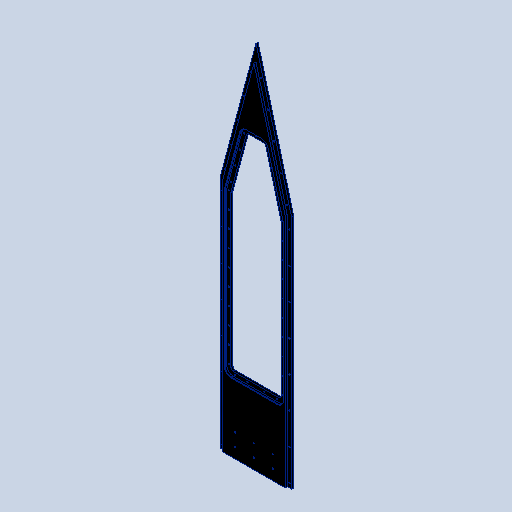
# Autodesk Inventor part: Model Shell_part1_side_plate
Saved by Autodesk Inventor 2023 (Build 270158000, 158)
## iProperties
Created: 2022-12-13
Part Number: Model Shell_part1_side_plate
Material: Aluminum 6061
Document SubType Name: Modeling
Designer: Tanzu
Density: 2.7 g/cm^3
Appearance: White
Mass: 6356.21 g
Surface Area: 9912.85 cm^2
Volume: 2354.15 cm^3
Author: Tanzu
Autodesk Inventor part; units mm, degrees
(part 1 of 2)
ref_plane "YZ Plane" through (0, 0, 0) normal (1, 0, 0) x (0, 1, 0)
ref_plane "XZ Plane" through (0, 0, 0) normal (0, 1, 0) x (-1, 0, 0)
ref_plane "XY Plane" through (0, 0, 0) normal (0, 0, 1) x (1, 0, 0)
sketch "Sketch2" plane through (0, 0, 0) normal (0, 0, 1) x (1, 0, 0)
  line L0 (-90, 0) -> (90, 0) construction
  line L1 (90, 0) -> (90, 900) construction
  line L2 (90, 900) -> (-90, 900) construction
  line L3 (-90, 900) -> (-90, 0) construction
  line L4 (-90, 250) -> (90, 250) construction
  line L5 (0, 900) -> (90, 564.1154)
  line L6 (0, 900) -> (-90, 564.1154)
  line L7 (0, 900) -> (0, 250) construction
  line L8 (-132.5, 0) -> (132.5, 0) construction
  line L9 (-90, 564.1154) -> (-90, 0)
  line L10 (90, 564.1154) -> (90, 0)
  line L11 (90, 0) -> (-90, 0)
  line L12 (-85, 563.4572) -> (0, 880.6815)
  line L13 (0, 880.6815) -> (85, 563.4572)
  line L14 (85, 563.4572) -> (85, 5)
  line L15 (85, 5) -> (-85, 5)
  line L16 (-85, 5) -> (-85, 563.4572)
  line L17 (-85, 5) -> (-85, 0)
  line L18 (85, 5) -> (85, 0)
  line L19 (40, 731.3995) -> (-40, 731.3995)
  line L20 (90, 564.1154) -> (-90, 564.1154) construction
  line L21 (85, 563.4572) -> (85, 564.1154)
  line L22 (85, 564.1154) -> (84.8236, 564.1154)
  line L23 (-85, 563.4572) -> (-85, 564.1154)
  line L24 (-85, 564.1154) -> (-84.8236, 564.1154)
  point P0 (0, 0)
  point P1 (0, 0)
  dimension "d4" = 180
  dimension "d5" = 900
  dimension "d6" = 250
  dimension "d7" = 15
  dimension "d8" = 15
  dimension "d9" = 265
  dimension "d10" = 5
  dimension "d265" = 80
  constraints: 50 end point, 15 point on line, 6 perpendicular, 4 midpoint, 3 coincident, 3 collinear, 2 horizontal, 2 parallel, 4 other
  measures "d4" distance of L0.start L0.end
  measures "d5" distance of L0.end L1.end
  measures "d6" distance between parallel lines of L0 L4
  measures "d7" angle of L7 L5
  measures "d8" angle of L6 L7
  measures "d9" distance of L8.start L8.end
  measures "d10" distance between parallel lines of L6 L12
  measures "d265" distance of L19.start L19.end
extrude "Extrusion2" add sketch "Sketch2" along normal mid plane 180
sketch "Sketch3" plane through (0, 0, 0) normal (0, 0, 1) x (1, 0, 0)
  line L0 (-132.5, 0) -> (132.5, 0)
  line L1 (-90, 0) -> (90, 0) projected
  line L2 (0, 0) -> (0, 600)
  line L3 (0, 600) -> (-132.5, 0)
  line L4 (0, 601.0824) -> (0, 600)
  line L5 (0, 577.3585) -> (-127.5, 0)
  line L6 (0, 577.3585) -> (0, 601.0824)
  point P0 (0, 0)
  dimension "d13" = 265
  dimension "d14" = 600
  dimension "d17" = 5
  constraints: 12 end point, 3 point on line, 2 midpoint, 2 vertical, 1 collinear, 1 horizontal, 1 parallel
  measures "d13" distance of L0.start L0.end
  measures "d14" distance of L2.start L2.end
  measures "d17" distance of L0.start L5.end
revolve "Revolution1" [suppressed]
revolve "Revolution2" [suppressed]
extrude "Extrusion3" cut sketch "Sketch2" along normal mid plane 160 contours L11 L17 L15 L18 | L15 L16 L12 L19 L13 L14 | L13 L22 L21 | L23 L24 L12 | L19 L12 L13
sketch "Sketch5" plane through (0, 0, 0) normal (0, -1, 0) x (1, 0, 0)
  circle A0 centre (0, 0) radius 127.5 projected
  circle A1 centre (0, 0) radius 132.5 projected
extrude "Extrusion4" [suppressed]
fillet "Fillet1" [suppressed]
sketch "Sketch6" plane through (90, 564.1154, 90) normal (1, 0, 0) x (0, 0, -1)
  line L0 (180, 0) -> (180, -564.1154) projected
  line L1 (180, 0) -> (0, 0) projected
  line L2 (0, -564.1154) -> (0, 0) projected
  line L3 (27.5, -275) -> (152.5, -275)
  line L4 (152.5, -275) -> (152.5, -75)
  line L5 (152.5, -75) -> (27.5, -75)
  line L6 (27.5, -75) -> (27.5, -275)
  line L7 (180, -564.1154) -> (0, -564.1154) projected
  point P0 (90, -564.1154)
  point P1 (90, 0)
  point P2 (90, -75)
  dimension "d25" = 75
  dimension "d26" = 200
  dimension "d27" = 125
  constraints: 8 end point, 2 midpoint, 2 parallel, 1 horizontal, 1 perpendicular, 1 vertical alignment
  measures "d25" distance between parallel lines of L1 L5
  measures "d26" distance of L5.end L3.start
  measures "d27" distance of L3.start L3.end
extrude "Extrusion5" cut sketch "Sketch6" against normal up to next contours L6 L5 L4 L3
sketch "Sketch7" plane through (85, 33.0197, 85) normal (-1, 0, 0) x (0, 0, 1)
  line L0 (-22.5, 256.0957) -> (-22.5, 456.0957) projected
  line L1 (-147.5, 256.0957) -> (-22.5, 256.0957) projected
  line L2 (-147.5, 456.0957) -> (-147.5, 256.0957) projected
  line L3 (-22.5, 456.0957) -> (-147.5, 456.0957) projected
  line L4 (-32.5, 446.0957) -> (-32.5, 266.0957)
  line L5 (-32.5, 266.0957) -> (-137.5, 266.0957)
  line L6 (-137.5, 266.0957) -> (-137.5, 446.0957)
  line L7 (-137.5, 446.0957) -> (-32.5, 446.0957)
  point P0 (-85, -33.0197)
  dimension "d30" = 10
  constraints: 8 end point, 3 other
  measures "d30" distance between parallel lines of L0 L4
extrude "Extrusion6" [suppressed]
fillet "Fillet3" radius 5 4 edges at (87.5, 289.1154, 62.5) (87.5, 289.1154, -62.5) (87.5, 489.1154, 62.5) (87.5, 489.1154, -62.5)
sketch "Sketch8" plane through (0, 0, -90) normal (0, 0, -1) x (-1, 0, 0)
  line L0 (90, 0) -> (90, 564.1154) projected
  line L1 (90, 564.1154) -> (0, 900) projected
  line L2 (0, 900) -> (-90, 564.1154) projected
  line L3 (-90, 564.1154) -> (-90, 0) projected
  line L4 (-90, 564.1154) -> (0, 900) projected
  line L5 (-20.0962, 825) -> (20.0962, 825)
  line L6 (0, 900) -> (90, 564.1154) projected
  line L7 (-90, 0) -> (90, 0) projected
  point P0 (0, 0)
  point P1 (20.0962, 825)
  dimension "d34" = 75
  constraints: 2 end point, 2 point on line, 1 horizontal
  measures "d34" distance from line of L1.end L5
extrude "Extrusion7" [suppressed]
sketch "Sketch9" plane through (0, 0, -90) normal (0, 0, -1) x (-1, 0, 0)
  line L0 (0, 900) -> (-90, 564.1154) projected
  line L1 (-90, 564.1154) -> (-90, 0) projected
  line L2 (90, 0) -> (90, 564.1154) projected
  line L3 (90, 564.1154) -> (0, 900) projected
  line L4 (-55, 164.1154) -> (55, 164.1154)
  line L5 (70, 179.1154) -> (70, 542.1406)
  line L6 (70, 544.1154) -> (-70, 544.1154) construction
  line L7 (-70, 542.1406) -> (-70, 179.1154)
  line L8 (-69.4889, 546.0229) -> (-32.7866, 682.9977)
  line L9 (-18.2977, 694.1154) -> (18.2977, 694.1154)
  line L10 (-90, 0) -> (-90, 564.1154) projected
  line L11 (32.7866, 682.9977) -> (69.4889, 546.0229)
  line L12 (-20.0962, 825) -> (-90, 564.1154) projected
  line L13 (90, 564.1154) -> (20.0962, 825) projected
  arc A0 (-70, 179.1154) -> (-55, 164.1154) centre (-55, 179.1154) ccw
  arc A1 (55, 164.1154) -> (70, 179.1154) centre (55, 179.1154) ccw
  arc A2 (-18.2977, 694.1154) -> (-32.7866, 682.9977) centre (-18.2977, 679.1154) ccw
  arc A3 (32.7866, 682.9977) -> (18.2977, 694.1154) centre (18.2977, 679.1154) ccw
  arc A4 (-69.4889, 546.0229) -> (-70, 542.1406) centre (-55, 542.1406) ccw
  arc A5 (70, 542.1406) -> (69.4889, 546.0229) centre (55, 542.1406) ccw
  line L14 (70, 542.1406) -> (70, 544.1154) construction
  line L15 (70, 544.1154) -> (69.4889, 546.0229) construction
  line L16 (-70, 542.1406) -> (-70, 544.1154) construction
  line L17 (-69.4889, 546.0229) -> (-70, 544.1154) construction
  line L18 (-65, 179.1154) -> (-65, 542.1406) construction
  arc A6 (-64.6593, 544.7288) -> (-65, 542.1406) centre (-55, 542.1406) ccw construction
  line L19 (-64.6593, 544.7288) -> (-27.957, 681.7036) construction
  arc A7 (-18.2977, 689.1154) -> (-27.957, 681.7036) centre (-18.2977, 679.1154) ccw construction
  line L20 (-18.2977, 689.1154) -> (18.2977, 689.1154) construction
  arc A8 (27.957, 681.7036) -> (18.2977, 689.1154) centre (18.2977, 679.1154) ccw construction
  line L21 (27.957, 681.7036) -> (64.6593, 544.7288) construction
  arc A9 (65, 542.1406) -> (64.6593, 544.7288) centre (55, 542.1406) ccw construction
  line L22 (65, 542.1406) -> (65, 179.1154) construction
  arc A10 (55, 169.1154) -> (65, 179.1154) centre (55, 179.1154) ccw construction
  line L23 (55, 169.1154) -> (-55, 169.1154) construction
  arc A11 (-65, 179.1154) -> (-55, 169.1154) centre (-55, 179.1154) ccw construction
  line L24 (-60, 542.1406) -> (-60, 179.1154)
  arc A12 (-60, 179.1154) -> (-55, 174.1154) centre (-55, 179.1154) ccw
  line L25 (-55, 174.1154) -> (55, 174.1154)
  arc A13 (55, 174.1154) -> (60, 179.1154) centre (55, 179.1154) ccw
  line L26 (60, 179.1154) -> (60, 542.1406)
  arc A14 (60, 542.1406) -> (59.8296, 543.4347) centre (55, 542.1406) ccw
  line L27 (59.8296, 543.4347) -> (23.1273, 680.4095)
  arc A15 (23.1273, 680.4095) -> (18.2977, 684.1154) centre (18.2977, 679.1154) ccw
  line L28 (18.2977, 684.1154) -> (-18.2977, 684.1154)
  arc A16 (-18.2977, 684.1154) -> (-23.1273, 680.4095) centre (-18.2977, 679.1154) ccw
  line L29 (-23.1273, 680.4095) -> (-59.8296, 543.4347)
  arc A17 (-59.8296, 543.4347) -> (-60, 542.1406) centre (-55, 542.1406) ccw
  circle A18 centre (-65, 184.1154) radius 1.5
  circle A19 centre (65, 184.1154) radius 1.5
  circle A20 centre (-65, 224.1154) radius 1.5
  circle A21 centre (65, 224.1154) radius 1.5
  circle A22 centre (-65, 264.1154) radius 1.5
  circle A23 centre (65, 264.1154) radius 1.5
  circle A24 centre (-65, 304.1154) radius 1.5
  circle A25 centre (65, 304.1154) radius 1.5
  circle A26 centre (-65, 344.1154) radius 1.5
  circle A27 centre (65, 344.1154) radius 1.5
  circle A28 centre (-65, 384.1154) radius 1.5
  circle A29 centre (65, 384.1154) radius 1.5
  circle A30 centre (-65, 424.1154) radius 1.5
  circle A31 centre (65, 424.1154) radius 1.5
  circle A32 centre (-65, 464.1154) radius 1.5
  circle A33 centre (65, 464.1154) radius 1.5
  circle A34 centre (-50, 169.1154) radius 1.5
  circle A35 centre (-20, 169.1154) radius 1.5
  circle A36 centre (-59.4646, 564.1154) radius 1.5
  circle A37 centre (-49.1119, 602.7525) radius 1.5
  circle A38 centre (-38.7591, 641.3895) radius 1.5
  circle A39 centre (-28.4063, 680.0265) radius 1.5
  circle A40 centre (0, 689.1154) radius 1.5
  line L30 (0, 164.1154) -> (0, 174.1154) construction
  circle A41 centre (50, 169.1154) radius 1.5
  circle A42 centre (20, 169.1154) radius 1.5
  circle A43 centre (59.4646, 564.1154) radius 1.5
  circle A44 centre (49.1119, 602.7525) radius 1.5
  circle A45 centre (38.7591, 641.3895) radius 1.5
  circle A46 centre (28.4063, 680.0265) radius 1.5
  line L31 (-90, 0) -> (90, 0) projected
  circle A47 centre (-65, 504.1154) radius 1.5
  circle A48 centre (65, 504.1154) radius 1.5
  circle A49 centre (-65, 544.1154) radius 1.5
  circle A50 centre (65, 544.1154) radius 1.5
  point P0 (0, 0)
  point P1 (-90, 37.1533)
  dimension "d37" = 20
  dimension "d38" = 20
  dimension "d39" = 20
  dimension "d41" = 150
  dimension "d42" = 15
  dimension "d43" = 15
  dimension "d44" = 15
  dimension "d45" = 15
  dimension "d46" = 15
  dimension "d47" = 15
  dimension "d48" = 380
  dimension "d49" = 5
  dimension "d50" = 5
  dimension "d51" = 3
  dimension "d52" = 3
  dimension "d53" = 10
  dimension "d59" = 40
  dimension "d63" = 3
  dimension "d64" = 15
  dimension "d70" = 30
  dimension "d72" = 3
  dimension "d79" = 40
  dimension "d81" = 3
  dimension "d721" = 20
  constraints: 51 centre point, 48 end point, 36 point on circle, 14 tangent, 6 parallel, 6 symmetric about line, 4 perpendicular, 4 point on line, 3 midpoint, 3 vertical, 2 horizontal, 1 collinear, 1 horizontal alignment, 73 other
  measures "d37" distance between parallel lines of L1 L7
  measures "d38" distance between parallel lines of L2 L5
  measures "d39" distance from line of L0.end L6
  measures "d41" distance between parallel lines of L6 L9
  measures "d42" radius of A1
  measures "d43" radius of A0
  measures "d44" radius of A4
  measures "d45" radius of A5
  measures "d46" radius of A2
  measures "d47" radius of A3
  measures "d48" distance between parallel lines of L6 L4
  measures "d49" distance between parallel lines of L7 L18
  measures "d50" distance between parallel lines of L24 L18
  measures "d51" diameter of A18
  measures "d52" diameter of A19
  measures "d53" distance from line of A18.centre L25
  measures "d59" distance of A18.centre A20.centre
  measures "d63" diameter of A34
  measures "d64" distance from line of L18 A34.centre
  measures "d70" distance of A34.centre A35.centre
  measures "d72" diameter of A36
  measures "d79" distance of A36.centre A37.centre
  measures "d81" diameter of A40
  measures "d721" vertical distance of A49.centre A36.centre
extrude "Extrusion8" cut sketch "Sketch9" against normal up to next contours A17 L29 A16 L28 A15 L27 A14 L26 A13 L25 A12 L24 | A18 | A19 | A20 | A21 | A22 | A23 | A24 | A25 | A26 | A27 | A28 | A29 | A30 | A31 | A32 | A33 | A34 | A35 | A36 | A37 | A38 | A39 | A40 | A41 | A42 | A43 | A44 | A45 | A46 | A47 | A48 | A49 | A50
extrude "Extrusion9" cut sketch "Sketch9" against normal blind 5 contours A0 L7 A4 L8 A2 L9 A3 L11 A5 L5 A1 L4 | A47 | A48 | A49 | A50
mirror "Mirror1" about plane through (0, 0, 0) normal (0, 0, 1) of "Extrusion8", "Extrusion9"
sketch "Sketch28" plane through (90, 0, 90) normal (1, 0, 0) x (0, 0, -1)
  arc A0 (147.5, 289.1154) -> (152.5, 294.1154) centre (147.5, 294.1154) ccw projected
  line L0 (147.5, 289.1154) -> (32.5, 289.1154) projected
  line L1 (152.5, 484.1154) -> (152.5, 294.1154) projected
  line L2 (32.5, 489.1154) -> (147.5, 489.1154) projected
  arc A1 (152.5, 484.1154) -> (147.5, 489.1154) centre (147.5, 484.1154) ccw projected
  line L3 (27.5, 294.1154) -> (27.5, 484.1154) projected
  arc A2 (32.5, 489.1154) -> (27.5, 484.1154) centre (32.5, 484.1154) ccw projected
  arc A3 (27.5, 294.1154) -> (32.5, 289.1154) centre (32.5, 294.1154) ccw projected
  line L4 (29.5, 484.1154) -> (29.5, 294.1154)
  arc A4 (29.5, 294.1154) -> (32.5, 291.1154) centre (32.5, 294.1154) ccw
  line L5 (32.5, 291.1154) -> (147.5, 291.1154)
  arc A5 (147.5, 291.1154) -> (150.5, 294.1154) centre (147.5, 294.1154) ccw
  line L6 (150.5, 294.1154) -> (150.5, 484.1154)
  arc A6 (150.5, 484.1154) -> (147.5, 487.1154) centre (147.5, 484.1154) ccw
  line L7 (147.5, 487.1154) -> (32.5, 487.1154)
  arc A7 (32.5, 487.1154) -> (29.5, 484.1154) centre (32.5, 484.1154) ccw
  point P0 (90, 0)
  dimension "d386" = 2
  constraints: 8 end point, 8 point on circle, 4 centre point, 7 other
  measures "d386" radial gap between concentric circles of A2 A7
extrude "Extrusion21" add sketch "Sketch28" along normal blind 2 from surface at -5
chamfer "Chamfer2" distance 1 angle 45 24 edges at (65.6066, 168.5088, -90) (70, 360.628, -90) (69.8717, 544.0985, -90) (51.1377, 614.5103, -90) (27.4291, 691.0157, -90) (0, 694.1154, -90) (-27.4291, 691.0157, -90) (-51.1377, 614.5103, -90) (-69.8717, 544.0985, -90) (-70, 360.628, -90) (-65.6066, 168.5088, -90) (0, 164.1154, -90) (0, 164.1154, 90) (-65.6066, 168.5088, 90) (-70, 360.628, 90) (-69.8717, 544.0985, 90) (-51.1377, 614.5103, 90) (-27.4291, 691.0157, 90) (0, 694.1154, 90) (27.4291, 691.0157, 90) (51.1377, 614.5103, 90) (69.8717, 544.0985, 90) (70, 360.628, 90) (65.6066, 168.5088, 90)
sketch "Sketch18" plane through (0, 0, 0) normal (0, 1, 0) x (-1, 0, 0)
  line L0 (-85, 80) -> (85, 80)
  line L1 (85, 80) -> (85, -80)
  line L2 (85, -80) -> (-85, -80)
  line L3 (-85, -80) -> (-85, 80)
  line L4 (80, 75) -> (-80, 75) construction
  line L5 (-80, 75) -> (-80, -75) construction
  line L6 (-80, -75) -> (80, -75) construction
  line L7 (80, -75) -> (80, 75) construction
  line L8 (-80, 75) -> (80, -75) construction
  line L9 (80, 75) -> (-80, -75) construction
  line L10 (85, 0) -> (-85, 0) construction
  line L11 (0, 80) -> (0, -80) construction
  line L12 (75, -70.3125) -> (-74.6667, -70.3125)
  line L13 (-74.6667, -70.3125) -> (-74.6667, 70)
  line L14 (-74.6667, 70) -> (75, 70)
  line L15 (75, 70) -> (75, -70.3125)
  line L16 (74, -69.3125) -> (-73.6667, -69.3125)
  line L17 (-73.6667, -69.3125) -> (-73.6667, 69)
  line L18 (-73.6667, 69) -> (74, 69)
  line L19 (74, 69) -> (74, -69.3125)
  line L20 (-61.6667, -60.625) -> (57, -60.625) construction
  line L21 (60, -57.625) -> (60, 53.25) construction
  line L22 (57, 56.25) -> (-61.6667, 56.25) construction
  line L23 (-64.6667, 53.25) -> (-64.6667, -57.625) construction
  arc A0 (-64.6667, -57.625) -> (-61.6667, -60.625) centre (-61.6667, -57.625) ccw construction
  arc A1 (57, -60.625) -> (60, -57.625) centre (57, -57.625) ccw construction
  arc A2 (60, 53.25) -> (57, 56.25) centre (57, 53.25) ccw construction
  arc A3 (-61.6667, 56.25) -> (-64.6667, 53.25) centre (-61.6667, 53.25) ccw construction
  line L24 (20, -57.625) -> (20, 53.25)
  line L25 (17, -60.625) -> (-61.6667, -60.625)
  line L26 (-64.6667, -57.625) -> (-64.6667, 53.25)
  line L27 (-61.6667, 56.25) -> (17, 56.25)
  arc A4 (17, -60.625) -> (20, -57.625) centre (17, -57.625) ccw
  arc A5 (20, 53.25) -> (17, 56.25) centre (17, 53.25) ccw
  arc A6 (-61.6667, 56.25) -> (-64.6667, 53.25) centre (-61.6667, 53.25) ccw
  arc A7 (-64.6667, -57.625) -> (-61.6667, -60.625) centre (-61.6667, -57.625) ccw
  point P0 (-64.6667, -60.625)
  point P1 (60, 56.25)
  point P2 (20, -60.625)
  point P3 (20, 56.25)
  dimension "d216" = 5
  dimension "d324" = 10
  dimension "d334" = 1
  dimension "d370" = 25
  dimension "d371" = 3
  dimension "d373" = 3
  dimension "d411" = 10
  dimension "d412" = 10
  dimension "d413" = 40
  constraints: 56 end point, 16 point on circle, 16 point on line, 16 tangent, 10 parallel, 8 centre point, 7 perpendicular, 6 equal radius, 4 midpoint, 3 horizontal, 2 coincident, 1 collinear, 1 vertical, 6 other
  measures "d216" distance between parallel lines of L0 L4
  measures "d324" distance between parallel lines of L0 L14
  measures "d334" distance between parallel lines of L15 L19
  measures "d370" distance between parallel lines of L1 L21
  measures "d371" radius of A0
  measures "d373" radius of A4
  measures "d411" distance between parallel lines of L1 L15
  measures "d412" distance between parallel lines of L13 L26
  measures "d413" distance between parallel lines of L21 L24
ref_plane "Work Plane15" through (-90, 180, -90) normal (0, -1, 0) x (1, 0, 0)
extrude "Extrusion12" add sketch "Sketch18" along normal blind 10 from surface at 180 separate body contours L0 L1 L2 L3 | L12 L13 L14 L15 | L16 L17 L18 L19 | A4 L25 A7 L26 A6 L27 A5 L24
extrude "Extrusion13" cut sketch "Sketch18" along normal through all contours A4 L25 A7 L26 A6 L27 A5 L24 bodies 2
extrude "Extrusion18" cut sketch "Sketch18" along normal blind 4 from surface at 180 contours L12 L13 L14 L15 | L16 L17 L18 L19 | A4 L25 A7 L26 A6 L27 A5 L24 bodies 2
extrude "Extrusion19" add sketch "Sketch18" along normal blind 3 from surface at 180 separate body contours L16 L17 L18 L19 | A4 L25 A7 L26 A6 L27 A5 L24
ref_plane "Work Plane10" through (90, 564.1154, 90) normal (0, -1, 0) x (1, 0, 0)
ref_plane "Work Plane11" through (0, 0, -80) normal (-1, 0, 0) x (0, 0, 1)
sketch "Sketch30" plane through (-90, 0, -90) normal (0, -1, 0) x (1, 0, 0)
  line L0 (175, 10) -> (175, 170) projected
  line L1 (175, 170) -> (175, 175)
  line L2 (175, 175) -> (165, 175)
  line L3 (165, 175) -> (165, 180)
  line L4 (180, 180) -> (90, 180) projected
  line L5 (5, 10) -> (5, 170) projected
  line L6 (5, 170) -> (5, 175)
  line L7 (5, 175) -> (15, 175)
  line L8 (15, 175) -> (15, 180)
  line L9 (0, 180) -> (180, 180) projected
  line L10 (5, 10) -> (5.1764, 10) projected
  line L11 (5, 10) -> (5, 5)
  line L12 (5, 5) -> (15, 5)
  line L13 (15, 5) -> (15, 0)
  line L14 (0, 0) -> (90, 0) projected
  line L15 (175, 10) -> (175, 5)
  line L16 (175, 5) -> (165, 5)
  line L17 (165, 5) -> (165, 0)
  line L18 (90, 0) -> (180, 0) projected
  line L19 (175, 170) -> (175, 10)
  line L20 (165, 0) -> (15, 0)
  line L21 (180, 0) -> (0, 0) projected
  line L22 (165, 180) -> (15, 180)
  point P0 (90, 90)
  dimension "d397" = 5
  dimension "d398" = 10
  dimension "d399" = 5
  dimension "d400" = 10
  dimension "d401" = 5
  dimension "d402" = 10
  dimension "d403" = 5
  dimension "d404" = 10
  constraints: 30 end point, 7 point on line, 6 perpendicular, 3 vertical, 2 collinear
  measures "d397" distance of L0.end L1.end
  measures "d398" distance of L1.end L2.end
  measures "d399" distance of L5.end L6.end
  measures "d400" distance of L6.end L7.end
  measures "d401" distance of L5.start L11.end
  measures "d402" distance of L11.end L12.end
  measures "d403" distance of L0.start L15.end
  measures "d404" distance of L15.end L16.end
ref_plane "Work Plane12" through (90, 564.1154, 0) normal (-0.258819, 0.9659258, 0) x (0, 0, 1)
sketch "Sketch31" plane through (90, 564.1154, 0) normal (-0.258819, 0.9659258, 0) x (0, 0, 1)
  line L0 (-90, 0) -> (90, 0) projected
  line L1 (90, 0) -> (-90, 0)
  line L2 (-90, 0) -> (-90, -15)
  line L3 (-90, -173.8666) -> (-90, 0) projected
  line L4 (-90, -15) -> (-85, -15)
  line L5 (-80, -168.8666) -> (-80, -5) projected
  line L6 (-85, -15) -> (-85, -5)
  line L7 (-85, -5) -> (85, -5)
  line L8 (-80, -4.8296) -> (80, -4.8296) projected
  line L9 (85, -5) -> (85, -15)
  line L10 (85, -15) -> (90, -15)
  line L11 (90, -15) -> (90, 0)
  point P0 (0, -232.9371)
  dimension "d406" = 15
  dimension "d407" = 5
  dimension "d408" = 10
  dimension "d409" = 10
  dimension "d410" = 5
  constraints: 16 end point, 3 perpendicular, 2 parallel, 1 collinear, 1 point on line, 1 vertical
  measures "d406" distance of L0.start L2.end
  measures "d407" distance of L2.end L4.end
  measures "d408" distance of L4.end L6.end
  measures "d409" distance of L7.end L9.end
  measures "d410" distance of L9.end L10.end
ref_plane "Work Plane13" through (-90, 564.1154, 0) normal (-0.258819, -0.9659258, 0) x (0, 0, 1)
sketch "Sketch32" plane through (-90, 564.1154, 0) normal (-0.258819, -0.9659258, 0) x (0, 0, 1)
  line L0 (-90, 0) -> (90, 0) projected
  line L1 (-90, 0) -> (-90, -15)
  line L2 (-90, -15) -> (-85, -15)
  line L3 (-85, -15) -> (-85, -5)
  line L4 (-85, -5) -> (85, -5)
  line L5 (80, -168.8666) -> (80, -5) projected
  line L6 (85, -5) -> (85, -15)
  line L7 (85, -15) -> (90, -15)
  line L8 (90, 0) -> (90, -146.0038) projected
  line L9 (90, -15) -> (90, 0)
  point P0 (0, -232.9371)
  dimension "d415" = 15
  dimension "d416" = 5
  dimension "d417" = 10
  dimension "d418" = 10
  dimension "d419" = 5
  constraints: 14 end point, 3 perpendicular, 2 point on line, 2 vertical
  measures "d415" distance of L0.start L1.end
  measures "d416" distance of L1.end L2.end
  measures "d417" distance of L2.end L3.end
  measures "d418" distance of L4.end L6.end
  measures "d419" distance of L6.end L7.end
split body "Split4" result two bodies by plane through (90, 564.1154, 90) normal (0, -1, 0) bodies 1 first body at (-89.5, 376.077, 30)
split body "Split5" result two bodies by plane through (0, 0, -80) normal (-1, 0, 0) bodies 5 first body at (-29.517, 787.9091, 30)
split body "Split6" sketch "Sketch32" result two bodies bodies 6 curves L1 L2 L3 L4 L6 L7 L9 L0 first body at (-29.517, 787.9091, 30)
split body "Split7" sketch "Sketch31" result two bodies bodies 7 curves L7 L9 L10 L11 L1 L2 L4 L6 first body at (59.517, 675.9475, -30)
split body "Split8" sketch "Sketch30" result two bodies bodies 4 curves L12 L13 L20 L17 L16 L15 L19 L1 L2 L3 L22 L8 L7 L6 L5 L11 first body at (6.6064, 55.8755, 80.5) (6.6064, 55.8755, -80.5)
combine bodies "Combine2" operation type add bodies to combine 9 11 12
sketch "Sketch33" plane through (0, 0, -90) normal (0, 0, -1) x (-1, 0, 0)
  line L0 (-90, 564.1154) -> (-90, 0) projected
  line L1 (-75, 0) -> (-75, 564.1154) projected
  line L2 (-90, 0) -> (-75, 0) projected
  point P0 (0, 0)
  point P1 (-80, 10)
  dimension "d428" = 5
  dimension "d429" = 10
  measures "d428" distance from line of point (-80, 10) L1
  measures "d429" distance from line of L2 point (-80, 10)
hole "Hole9" at (80, 10, -90) direction (0, 0, 1) diameter 4 depth 5 tip angle 118 countersink diameter 8 countersink angle 90 bodies 13
pattern_linear "Rectangular Pattern3" count 8 spacing 75 along (0, 1, 0) count 2 spacing 160 along (-1, 0, 0) of "Hole9" bodies 13
mirror "Mirror6" about plane through (0, 0, 0) normal (0, 0, 1) of "Hole9", "Rectangular Pattern3" bodies 13
sketch "Sketch35" plane through (0, 0, -90) normal (0, 0, -1) x (-1, 0, 0)
  line L0 (-74.4709, 564.1154) -> (-84.8236, 564.1154) projected
  line L1 (-79.6472, 564.1154) -> (-74.4709, 583.4339)
  line L2 (0, 842.0445) -> (-74.4709, 564.1154) projected
  point P0 (0, 0)
  dimension "d484" = 20
  dimension "d485" = 5
  constraints: 2 end point, 1 coincident, 1 midpoint, 1 parallel
  measures "d484" distance of L1.start L1.end
  measures "d485" distance between parallel lines of L2 L1
hole "Hole10" at (74.4709, 583.4339, -90) direction (0, 0, 1) diameter 4 depth 5 tip angle 118 countersink diameter 8 countersink angle 90 bodies 10
pattern_linear "Rectangular Pattern4" count 5 spacing 60 along (-0.258819, 0.9659258, 0) of "Hole10" bodies 10
mirror "Mirror7" about plane through (0, 0, 0) normal (0, 0, 1) of "Hole10", "Rectangular Pattern4" bodies 10
mirror "Mirror8" about plane through (0, 0, 0) normal (1, 0, 0) of "Hole10", "Rectangular Pattern4", "Mirror7" bodies 10 8
sketch "Sketch36" plane through (85, 0, -85) normal (0, 0, -1) x (-1, 0, 0)
  line L0 (0, 564.1154) -> (0, 0) projected
  line L1 (0, 0) -> (10, 0) projected
  point P0 (85, 0)
  point P1 (5, 10)
  dimension "d465" = 5
  dimension "d466" = 10
  measures "d465" distance from line of L0 point (5, 10)
  measures "d466" distance from line of L1 point (5, 10)
hole "Hole11" at (80, 10, -85) direction (0, 0, 1) diameter 3.242 depth 11.8 tip angle 118 bodies 9
pattern_linear "Rectangular Pattern5" count 8 spacing 75 along (0, 1, 0) count 2 spacing 160 along (-1, 0, 0) of "Hole11" bodies 9
sketch "Sketch37" plane through (85, 0, -85) normal (0, 0, -1) x (-1, 0, 0)
  line L0 (0, 564.1154) -> (0, 0) construction
  line L1 (0, 564.1154) -> (4.9942, 562.7772) construction
  line L2 (4.9942, 562.7772) -> (87.5882, 871.0222) construction
  line L3 (85, 880.6815) -> (169.8236, 564.1154) construction
  line L4 (0.1764, 564.1154) -> (85, 880.6815) construction
  line L5 (85, 842.0445) -> (10.5291, 564.1154) projected
  line L6 (10.5291, 564.1154) -> (85, 842.0445) construction
  line L7 (0.1764, 564.1154) -> (85, 880.6815) construction
  line L8 (10.5291, 564.1154) -> (0.1764, 564.1154) construction
  line L9 (10.5291, 583.4339) -> (5.3528, 564.1154) construction
  point P0 (85, 0)
  dimension "d482" = 5
  dimension "d486" = 20
  constraints: 8 end point, 3 point on line, 1 horizontal, 1 midpoint, 1 parallel, 1 perpendicular
  measures "d482" distance between parallel lines of L5 L2
  measures "d486" distance of L9.start L9.end
hole "Hole12" at (74.4709, 583.4339, -85) direction (0, 0, 1) diameter 3.242 depth 11.8 tip angle 118 bodies 9
pattern_linear "Rectangular Pattern6" count 5 spacing 60 along (-0.258819, 0.9659258, 0) of "Hole12" bodies 9
mirror "Mirror9" about plane through (0, 0, 0) normal (1, 0, 0) of "Hole12", "Rectangular Pattern6" bodies 9
mirror "Mirror10" about plane through (0, 0, 0) normal (0, 0, 1) of "Hole12", "Rectangular Pattern6", "Mirror9", "Hole11", "Rectangular Pattern5" bodies 9
sketch "Sketch38" plane through (0, 0, 0) normal (0, 0, 1) x (1, 0, 0)
  line L0 (84.8236, 564.1154) -> (0, 880.6815) projected
  line L1 (35, 750.0597) -> (-35, 750.0597)
  line L2 (0, 880.6815) -> (-84.8236, 564.1154) projected
  line L3 (0, 880.6815) -> (0, 842.0445) projected
  line L4 (35, 750.0597) -> (0, 880.6815)
  line L5 (0, 880.6815) -> (-35, 750.0597)
  line L6 (0, 900) -> (-90, 564.1154) projected
  line L7 (2.5, 765.0597) -> (30.9808, 765.0597)
  line L8 (2.5, 823.0242) -> (2.5, 765.0597)
  line L9 (-2.5, 823.0242) -> (-2.5, 765.0597)
  line L10 (-2.5, 765.0597) -> (-30.9808, 765.0597)
  line L11 (0, 880.6815) -> (-84.8236, 564.1154) projected
  line L12 (90, 564.1154) -> (0, 900) projected
  line L13 (0, 900) -> (19.4114, 827.5556) construction
  line L14 (19.4114, 827.5556) -> (2.5, 823.0242)
  line L15 (0, 900) -> (-19.4114, 827.5556) construction
  line L16 (-19.4114, 827.5556) -> (-2.5, 823.0242)
  point P0 (0, 0)
  point P1 (-14.5818, 826.2615)
  point P2 (14.5818, 826.2615)
  dimension "d490" = 70
  dimension "d492" = 5
  dimension "d494" = 15
  dimension "d501" = 75
  dimension "d502" = 75
  constraints: 22 end point, 7 point on line, 3 perpendicular, 2 vertical, 1 collinear, 1 horizontal, 1 parallel
  measures "d490" distance of L1.start L1.end
  measures "d492" distance between parallel lines of L9 L8
  measures "d494" distance between parallel lines of L1 L7
  measures "d501" distance of L6.start L13.end
  measures "d502" distance of L6.start L15.end
extrude "Extrusion22" add sketch "Sketch38" along normal mid plane 160 separate body contours L1 L2 L10 L9 L16 L0 L14 L8 L7 | L7 L8 L14 L0 | L2 L16 L9 L10
extrude "Extrusion23" cut sketch "Sketch38" along normal mid plane 150 contours L1 L2 L10 L9 L16 L0 L14 L8 L7 | L7 L8 L14 L0 | L2 L16 L9 L10 bodies 14
extrude "Extrusion24" cut sketch "Sketch38" along normal mid plane 160 contours L7 L8 L14 L0 | L2 L16 L9 L10 bodies 14
sketch "Sketch39" plane through (-35, 750.0597, 80) normal (0, -1, 0) x (1, 0, 0)
  line L0 (35, -165) -> (35, 5) projected
  line L1 (42.5, 0) -> (27.5, 0)
  line L2 (27.5, 0) -> (27.5, -160)
  line L3 (27.5, -160) -> (42.5, -160)
  line L4 (42.5, -160) -> (42.5, 0)
  line L5 (0, 0) -> (70, 0) projected
  line L6 (70, -160) -> (0, -160) projected
  line L7 (42.5, -4.5) -> (27.5, -4.5)
  line L8 (42.5, -155.5) -> (27.5, -155.5)
  line L9 (35, -170) -> (35, 10) projected
  line L10 (35, 0) -> (35, -53.3333) construction
  line L11 (35, -53.3333) -> (35, -106.6667) construction
  line L12 (35, -106.6667) -> (35, -160) construction
  point P0 (35, -80)
  dimension "d503" = 15
  dimension "d504" = 7.5
  dimension "d505" = 4.5
  dimension "d506" = 4.5
  constraints: 18 end point, 4 midpoint, 4 point on line, 3 equal length, 3 perpendicular, 2 coincident, 2 collinear, 1 horizontal, 3 other
  measures "d503" distance between parallel lines of L2 L4
  measures "d504" distance between parallel lines of L4 L0
  measures "d505" distance between parallel lines of L5 L7
  measures "d506" distance between parallel lines of L6 L8
extrude "Extrusion25" add sketch "Sketch39" against normal blind 5 separate body contours L8 L2 L7 L0 | L0 L7 L4 L8
extrude "Extrusion26" add sketch "Sketch39" against normal blind 3 contours L3 L2 L8 L0 | L0 L8 L4 L3 | L7 L2 L1 L0 | L0 L1 L4 L7 bodies 15
extrude "Extrusion27" cut sketch "Sketch39" against normal blind 5 contours L8 L2 L7 L0 | L0 L7 L4 L8 bodies 14
extrude "Extrusion28" cut sketch "Sketch39" against normal blind 3 contours L3 L2 L8 L0 | L0 L8 L4 L3 | L7 L2 L1 L0 | L0 L1 L4 L7 bodies 14
sketch "Sketch40" plane through (2.5, 765.0597, 75) normal (1, 0, 0) x (0, 0, -1)
  line L0 (-5, 0) -> (-5, 57.9645) projected
  line L1 (155, 0) -> (155, 57.9645) projected
  line L2 (-5, 42.9645) -> (155, 42.9645)
  line L3 (155, 42.9645) -> (155, 32.9645)
  line L4 (155, 32.9645) -> (-5, 32.9645)
  line L5 (-5, 32.9645) -> (-5, 42.9645)
  line L6 (0, 57.9645) -> (-5, 57.9645) projected
  line L7 (0, 57.9645) -> (0, 0) projected
  line L8 (0, 42.9645) -> (0, 32.9645)
  line L9 (150, 57.9645) -> (150, 0) projected
  line L10 (150, 42.9645) -> (150, 32.9645)
  point P0 (75, -765.0597)
  point P1 (-5, 37.9645)
  point P2 (-5, 32.9645)
  point P3 (155, 42.9645)
  dimension "d515" = 20
  dimension "d516" = 10
  constraints: 12 end point, 10 point on line, 2 parallel, 1 horizontal, 1 midpoint, 1 perpendicular
  measures "d515" distance from line of point (-5, 37.964) L6
  measures "d516" distance between parallel lines of L2 L4
extrude "Extrusion29" add sketch "Sketch40" against normal blind 2 separate body contours L7 L2 L9 L4
extrude "Extrusion30" add sketch "Sketch40" along normal blind 3 contours L0 L2 L7 L4 | L7 L2 L9 L4 | L9 L2 L1 L4 bodies 16
sketch "Sketch41" plane through (5.5, 765.0597, 75) normal (1, 0, 0) x (0, 0, -1)
  line L0 (155, 42.9645) -> (-5, 42.9645) projected
  line L1 (155, 32.9645) -> (155, 42.9645) projected
  line L2 (-5, 42.9645) -> (-5, 32.9645) projected
  point P0 (75, -765.0597)
  point P1 (-2, 37.9645)
  point P2 (152, 37.9645)
  dimension "d528" = 5
  dimension "d529" = 3
  dimension "d530" = 5
  dimension "d531" = 3
  measures "d528" distance from line of point (152, 37.964) L0
  measures "d529" distance from line of L1 point (152, 37.964)
  measures "d530" distance from line of L0 point (-2, 37.964)
  measures "d531" distance from line of L2 point (-2, 37.964)
hole "Hole13" at (5.5, 803.0242, 77) at (5.5, 803.0242, -77) direction (-1, 0, 0) diameter 3 depth 13.8 tip angle 118 counterbore diameter 5 counterbore depth 2 bodies 16
sketch "Sketch42" plane through (2.5, 765.0597, 75) normal (1, 0, 0) x (0, 0, -1)
  circle A0 centre (-2, 37.9645) radius 1.5 projected
  circle A1 centre (152, 37.9645) radius 1.5 projected
  point P0 (75, -765.0597)
  constraints: 2 coincident
hole "Hole14" at (2.5, 803.0242, 77) at (2.5, 803.0242, -77) direction (-1, 0, 0) diameter 2.459 depth 8.8 tip angle 118 bodies 14
sketch "Sketch43" plane through (-35, 750.0597, 80) normal (0, -1, 0) x (1, 0, 0)
  line L0 (27.5, 0) -> (27.5, -160) projected
  line L1 (27.5, -160) -> (42.5, -160) projected
  line L2 (42.5, 0) -> (27.5, 0) projected
  point P0 (35, -80)
  point P1 (35, -2.5)
  point P2 (35, -157.5)
  dimension "d546" = 7.5
  dimension "d547" = 2.5
  dimension "d548" = 7.5
  dimension "d549" = 2.5
  measures "d546" distance from line of L0 point (35, -157.5)
  measures "d547" distance from line of L1 point (35, -157.5)
  measures "d548" distance from line of L0 point (35, -2.5)
  measures "d549" distance from line of L2 point (35, -2.5)
hole "Hole15" at (0, 750.0597, 77.5) at (0, 750.0597, -77.5) direction (0, 1, 0) diameter 3 depth 8.8 tip angle 118 counterbore diameter 4 counterbore depth 2 bodies 15
sketch "Sketch44" plane through (-35, 753.0597, 80) normal (0, -1, 0) x (1, 0, 0)
  circle A0 centre (35, -157.5) radius 1.5 projected
  circle A1 centre (35, -2.5) radius 1.5 projected
  point P0 (35, -80)
  constraints: 2 coincident
hole "Hole16" at (0, 753.0597, 77.5) at (0, 753.0597, -77.5) direction (0, 1, 0) diameter 2.459 depth 8.8 tip angle 118 bodies 14
sketch "Sketch45" plane through (-35, 750.0597, 80) normal (0, -1, 0) x (1, 0, 0)
  line L0 (27.5, 0) -> (42.5, 0) construction
  line L1 (35, 0) -> (35, -160) construction
  line L2 (27.5, -160) -> (42.5, -160) construction
  line L3 (27.5, 0) -> (27.5, -160) construction
  point P0 (35, -80)
  point P1 (35, -60)
  point P2 (35, -100)
  dimension "d564" = 7.5
  dimension "d565" = 60
  dimension "d566" = 60
  constraints: 2 end point, 2 midpoint, 2 point on line, 1 vertical
  measures "d564" distance between parallel lines of L3 L1
  measures "d565" distance from line of point (35, -100) L2
  measures "d566" distance from line of L0 point (35, -60)
hole "Hole17" at (0, 750.0597, 20) at (0, 750.0597, -20) direction (0, 1, 0) diameter 2.459 depth 8.8 tip angle 118 bodies 15
sketch "Sketch46" plane through (-84.8236, 564.1154, 85) normal (0.9659258, -0.258819, 0) x (0, 0, -1)
  line L0 (10, 271.3936) -> (5, 271.3936) projected
  line L1 (165, 271.3936) -> (160, 271.3936) projected
  line L2 (5, 271.3936) -> (165, 271.3936)
  line L3 (165, 271.3936) -> (165, 268.3936)
  line L4 (165, 0) -> (165, 327.7333) projected
  line L5 (165, 268.3936) -> (5, 268.3936)
  line L6 (5, 327.7333) -> (5, 0) projected
  line L7 (5, 268.3936) -> (5, 271.3936)
  line L8 (160, 271.3936) -> (160, 327.7333) projected
  line L9 (160, 268.3936) -> (160, 271.3936)
  line L10 (164, 268.3936) -> (164, 271.3936)
  line L11 (6, 268.3936) -> (6, 271.3936)
  line L12 (10, 268.3936) -> (10, 271.3936)
  point P0 (85, -522.9397)
  point P1 (6, 269.8936)
  point P2 (6, 271.3936)
  dimension "d567" = 3
  dimension "d570" = 1
  dimension "d571" = 1
  constraints: 16 end point, 8 point on line, 5 perpendicular, 1 collinear, 1 horizontal, 1 midpoint
  measures "d567" distance of L1.start L3.end
  measures "d570" distance between parallel lines of L3 L10
  measures "d571" distance from line of point (6, 269.894) L7
extrude "Extrusion31" add sketch "Sketch46" along normal blind 2 contours L12 L5 L11 L0 | L1 L10 L5 L9 bodies 8
mirror "Mirror11" about plane through (0, 0, 0) normal (1, 0, 0) of "Extrusion31" bodies 10
sketch "Sketch47" plane through (0, 0, 80) normal (0, 0, 1) x (1, 0, 0)
  circle A0 centre (-27.8834, 757.3006) radius 2 projected
  circle A1 centre (27.8834, 757.3006) radius 2 projected
  circle A2 centre (27.8834, 757.3006) radius 2 projected
  point P0 (0, 0)
  constraints: 2 coincident
hole "Hole18" at (-27.8834, 757.3006, 80) at (27.8834, 757.3006, 80) direction (0, 0, -1) diameter 3.242 depth 11.8 tip angle 118 bodies 14
mirror "Mirror12" about plane through (0, 0, 0) normal (0, 0, 1) of "Hole18" bodies 14
sketch "Sketch48" plane through (0, 0, 0) normal (0, 0, 1) x (1, 0, 0)
  line L0 (-75, 184) -> (-65, 184)
  line L1 (-65, 184) -> (-65, 179) construction
  line L2 (-65, 179) -> (-75, 179)
  line L3 (-75, 179) -> (-75, 184)
  line L4 (73.6667, 180) -> (-74, 180) projected
  line L5 (-65, 179) -> (-65, 180)
  line L6 (85, 180) -> (-85, 180) projected
  line L7 (-74, 180) -> (-65, 180)
  line L8 (-74, 180) -> (-74, 183) projected
  line L9 (-74, 180) -> (-74, 183)
  line L10 (-74, 183) -> (-65, 183)
  line L11 (73.6667, 183) -> (-74, 183) projected
  line L12 (-65, 183) -> (-65, 184)
  line L13 (74.6667, 184) -> (-75, 184) projected
  point P0 (0, 0)
  dimension "d579" = 1
  dimension "d580" = 10
  constraints: 18 end point, 4 point on line, 2 collinear, 2 parallel, 2 perpendicular, 1 horizontal
  measures "d579" distance between parallel lines of L2 L4
  measures "d580" distance between parallel lines of L3 L1
sketch3d "3D Sketch3"
  line L0 (-74, 180, 69) -> (-74, 180, -69.3125)
  line L1 (-74, 180, -69.3125) -> (73.6667, 180, -69.3125)
  line L2 (73.6667, 180, -69.3125) -> (73.6667, 180, 69)
  line L3 (73.6667, 180, 69) -> (-74, 180, 69)
sweep "Sweep3" add profiles "Sketch48" path "3D Sketch3" separate body
sketch "Sketch49" plane through (-75, 179, -70.3125) normal (0, -1, 0) x (1, 0, 0)
  line L0 (139.6667, 130.3125) -> (10, 130.3125) projected
  line L1 (10, 130.3125) -> (10, 10) projected
  point P0 (75, 70.3125)
  point P1 (5, 135.3125)
  dimension "d590" = 5
  dimension "d591" = 5
  measures "d590" distance from line of L0 point (5, 135.313)
  measures "d591" distance from line of point (5, 135.313) L1
hole "Hole19" at (-70, 179, 65) direction (0, 1, 0) diameter 2.459 depth 8.8 tip angle 118 bodies 17 3
pattern_linear "Rectangular Pattern7" count 2 spacing 40 along (0, 0, -1) of "Hole19" bodies 17 3
pattern_linear "Rectangular Pattern8" count 2 spacing 40 along (1, 0, 0) of "Hole19" bodies 17 3
sketch "Sketch50" plane through (-75, 184, -70.3125) normal (0, -1, 0) x (1, 0, 0)
  circle A0 centre (5, 135.3125) radius 1.2295 projected
  circle A1 centre (5, 135.3125) radius 1.2295 projected
  circle A2 centre (5, 95.3125) radius 1.2295 projected
  circle A3 centre (5, 95.3125) radius 1.2295 projected
  circle A4 centre (45, 135.3125) radius 1.2295 projected
  point P0 (75, 70.3125)
  constraints: 3 coincident
hole "Hole20" at (-70, 184, 65) at (-30, 184, 65) at (-70, 184, 25) direction (0, 1, 0) diameter 2.459 depth 8.8 tip angle 118 bodies 2
mirror "Mirror13" about plane through (0, 0, 0) normal (0, 0, 1) of "Hole19", "Rectangular Pattern7", "Rectangular Pattern8", "Hole20" bodies 3 17 2
mirror "Mirror14" about plane through (0, 0, 0) normal (1, 0, 0) of "Hole19", "Rectangular Pattern7", "Rectangular Pattern8", "Mirror13", "Hole20" bodies 3 17 2
sketch "Sketch51" plane through (-75, 184, -70.3125) normal (0, -1, 0) x (1, 0, 0)
  line L0 (-10, 150.3125) -> (160, 150.3125) projected
  line L1 (160, -9.6875) -> (-10, -9.6875) projected
  line L2 (-10, 150.3125) -> (160, 150.3125) projected
  line L3 (35, 150.3125) -> (35, -9.6875) construction
  line L4 (55, 12.6875) -> (55, 123.5625) projected
  point P0 (75, 70.3125)
  point P1 (35, 105.3125)
  point P2 (35, 70.3125)
  point P3 (35, 35.3125)
  dimension "d612" = 45
  dimension "d613" = 45
  dimension "d615" = 20
  dimension "d616" = 35
  constraints: 4 point on line, 2 end point, 1 midpoint, 1 perpendicular
  measures "d612" distance from line of L0 point (35, 105.313)
  measures "d613" distance from line of point (35, 35.313) L1
  measures "d615" distance between parallel lines of L4 L3
  measures "d616" distance of point (35, 35.313) point (35, 70.313)
hole "Hole21" at (-40, 184, 35) at (-40, 184, 0) at (-40, 184, -35) direction (0, 1, 0) diameter 3 depth 8.8 tip angle 118 counterbore diameter 5 counterbore depth 3 bodies 2
sketch "Sketch55" plane through (75, 0, -90) normal (0, 0, -1) x (-1, 0, 0)
  line L0 (-57.8002, 25) -> (178.7484, 25) construction
  line L1 (0, 0) -> (150, 0) construction
  line L2 (-15, 564.1154) -> (-15, 0) construction
  line L3 (-44.1029, 55) -> (178.7484, 55) construction
  line L4 (-49.5633, 100) -> (178.7484, 100) construction
  point P0 (75, 0)
  point P1 (30, 25)
  point P2 (75, 25)
  point P3 (120, 25)
  point P4 (30, 55)
  point P5 (75, 55)
  point P6 (120, 55)
  dimension "d647" = 25
  dimension "d648" = 45
  dimension "d649" = 45
  dimension "d650" = 45
  dimension "d697" = 30
  dimension "d698" = 45
  constraints: 6 end point, 6 point on line, 3 horizontal, 3 vertical alignment
  measures "d647" distance between parallel lines of L1 L0
  measures "d648" distance from line of point (30, 25) L2
  measures "d649" distance of point (30, 25) point (75, 25)
  measures "d650" distance of point (120, 25) point (75, 25)
  measures "d697" distance between parallel lines of L3 L0
  measures "d698" distance between parallel lines of L3 L4
hole "Hole24" at (45, 25, -90) at (0, 25, -90) at (-45, 25, -90) at (45, 55, -90) at (0, 55, -90) at (-45, 55, -90) direction (0, 0, 1) diameter 3.242 depth 11.8 tip angle 118 bodies 9
mirror "Mirror16" about plane through (0, 0, 0) normal (0, 0, 1) of "Hole24" bodies 9
ref_plane "Work Plane16" through (90, 0, 90) normal (-0.7071068, 0, 0.7071068) x (0, 1, 0)
mirror "Mirror17" about plane through (90, 0, 90) normal (-0.7071068, 0, 0.7071068) of "Hole24", "Mirror16" bodies 9 13
sketch "Sketch56" plane through (-85, 0, -80) normal (0, 0, 1) x (1, 0, 0)
  point P0 (165, 10)
  point P1 (165, 85)
  point P2 (165, 160)
  point P3 (165, 235)
  point P4 (165, 310)
  point P5 (165, 385)
  point P6 (165, 460)
  point P7 (165, 535)
  point P8 (5, 10)
  point P9 (5, 85)
  point P10 (5, 160)
  point P11 (5, 235)
  point P12 (5, 310)
  point P13 (5, 385)
  point P14 (5, 460)
  point P15 (5, 535)
hole "Hole25" at (80, 10, -80) at (80, 85, -80) at (80, 160, -80) at (80, 235, -80) at (80, 310, -80) at (80, 385, -80) at (80, 460, -80) at (80, 535, -80) at (-80, 10, -80) at (-80, 85, -80) at (-80, 160, -80) at (-80, 235, -80) at (-80, 310, -80) at (-80, 385, -80) at (-80, 460, -80) at (-80, 535, -80) direction (0, 0, -1) diameter 4.5 depth 5 bodies 9
sketch "Sketch57" plane through (90, 0, 90) normal (1, 0, 0) x (0, 0, -1)
  line L0 (8, 254.1154) -> (172, 254.1154)
  line L1 (175, 257.1154) -> (175, 511.1154)
  line L2 (172, 514.1154) -> (8, 514.1154)
  line L3 (5, 511.1154) -> (5, 257.1154)
  line L4 (180, 564.1154) -> (0, 564.1154) projected
  line L5 (180, 564.1154) -> (180, 0) projected
  line L6 (0, 0) -> (0, 564.1154) projected
  line L7 (162, 264.1154) -> (18, 264.1154)
  line L8 (15, 267.1154) -> (15, 501.1154)
  line L9 (18, 504.1154) -> (162, 504.1154)
  line L10 (165, 501.1154) -> (165, 267.1154)
  arc A0 (5, 257.1154) -> (8, 254.1154) centre (8, 257.1154) ccw
  arc A1 (15, 267.1154) -> (18, 264.1154) centre (18, 267.1154) ccw
  arc A2 (162, 264.1154) -> (165, 267.1154) centre (162, 267.1154) ccw
  arc A3 (172, 254.1154) -> (175, 257.1154) centre (172, 257.1154) ccw
  arc A4 (165, 501.1154) -> (162, 504.1154) centre (162, 501.1154) ccw
  arc A5 (175, 511.1154) -> (172, 514.1154) centre (172, 511.1154) ccw
  arc A6 (18, 504.1154) -> (15, 501.1154) centre (18, 501.1154) ccw
  arc A7 (8, 514.1154) -> (5, 511.1154) centre (8, 511.1154) ccw
  point P0 (90, 0)
  point P1 (5, 254.1154)
  point P2 (175, 514.1154)
  point P3 (5, 514.1154)
  dimension "d658" = 50
  dimension "d659" = 260
  dimension "d660" = 5
  dimension "d662" = 170
  dimension "d663" = 10
  dimension "d664" = 3
  constraints: 16 end point, 16 point on circle, 16 tangent, 8 centre point, 7 equal radius, 6 point on line, 4 parallel, 2 perpendicular, 1 horizontal, 3 other
  measures "d658" distance between parallel lines of L2 L4
  measures "d659" distance of point (5, 514.115) point (5, 254.115)
  measures "d660" distance between parallel lines of L5 L1
  measures "d662" distance of point (175, 514.115) point (5, 514.115)
  measures "d663" distance between parallel lines of L0 L7
  measures "d664" radius of A0
extrude "Extrusion33" cut sketch "Sketch57" against normal blind 10 contours L7 A1 L8 A6 L9 A4 L10 A2 bodies 13
extrude "Extrusion34" cut sketch "Sketch57" against normal blind 2 bodies 13
sketch "Sketch58" plane through (88, 0, 90) normal (1, 0, 0) x (0, 0, -1)
  line L0 (18, 264.1154) -> (162, 264.1154) projected
  line L1 (15, 501.1154) -> (15, 267.1154) projected
  line L2 (165, 267.1154) -> (165, 501.1154) projected
  point P0 (90, 0)
  point P1 (170, 259.1154)
  point P2 (10, 259.1154)
  dimension "d676" = 5
  dimension "d677" = 5
  dimension "d678" = 5
  dimension "d679" = 5
  measures "d676" distance from line of L0 point (10, 259.115)
  measures "d677" distance from line of point (10, 259.115) L1
  measures "d678" distance from line of point (170, 259.115) L0
  measures "d679" distance from line of point (170, 259.115) L2
hole "Hole26" at (88, 259.1154, -80) at (88, 259.1154, 80) direction (-1, 0, 0) diameter 3.242 depth 3 tip angle 118 bodies 13
pattern_linear "Rectangular Pattern9" count 7 spacing 50 along (0, 1, 0) of "Hole26" bodies 13
sketch "Sketch59" plane through (88, 0, 90) normal (1, 0, 0) x (0, 0, -1)
  circle A0 centre (170, 509.1154) radius 1.621 projected
  line L0 (162, 504.1154) -> (18, 504.1154) projected
  circle A1 centre (170, 259.1154) radius 1.621 projected
  line L1 (18, 264.1154) -> (162, 264.1154) projected
  point P0 (90, 0)
  point P1 (130, 259.1154)
  point P2 (130, 509.1154)
  dimension "d690" = 40
  dimension "d691" = 5
  dimension "d692" = 40
  dimension "d693" = 5
  measures "d690" distance of A0.centre point (130, 509.115)
  measures "d691" distance from line of L0 point (130, 509.115)
  measures "d692" distance of A1.centre point (130, 259.115)
  measures "d693" distance from line of L1 point (130, 259.115)
hole "Hole27" at (88, 259.1154, -40) at (88, 509.1154, -40) direction (-1, 0, 0) diameter 3.242 depth 3 tip angle 118 bodies 13
pattern_linear "Rectangular Pattern10" count 3 spacing 40 along (0, 0, 1) of "Hole27" bodies 13
sketch "Sketch60" plane through (85, 190, -80) normal (0, 0, -1) x (-1, 0, 0)
  line L0 (0, 0) -> (0, -10) construction
  line L1 (0, -5) -> (170, -5) construction
  line L2 (170, -10) -> (170, 0) construction
  line L3 (-5, 374.1154) -> (-5, -190) projected
  point P0 (85, -190)
  point P1 (40, -5)
  point P2 (85, -5)
  point P3 (130, -5)
  dimension "d706" = 45
  dimension "d707" = 45
  dimension "d708" = 45
  constraints: 3 midpoint, 2 end point, 2 point on line
  measures "d706" distance of point (40, -5) point (85, -5)
  measures "d707" distance of point (130, -5) point (85, -5)
  measures "d708" distance from line of point (40, -5) L3
hole "Hole28" at (45, 185, -80) at (0, 185, -80) at (-45, 185, -80) direction (0, 0, 1) diameter 3.242 depth 4 tip angle 118 bodies 2
sketch "Sketch61" plane through (-85, 190, 80) normal (0, 0, 1) x (1, 0, 0)
  line L0 (175, -190) -> (175, 374.1154) projected
  line L1 (170, -10) -> (170, 0) construction
  line L2 (170, -5) -> (0, -5) construction
  line L3 (0, -10) -> (0, 0) construction
  point P0 (85, -190)
  point P1 (130, -5)
  point P2 (85, -5)
  point P3 (40, -5)
  dimension "d716" = 45
  dimension "d717" = 45
  dimension "d718" = 45
  constraints: 3 midpoint, 2 end point, 2 point on line
  measures "d716" distance from line of point (130, -5) L0
  measures "d717" distance of point (85, -5) point (130, -5)
  measures "d718" distance of point (40, -5) point (85, -5)
hole "Hole29" at (45, 185, 80) at (0, 185, 80) at (-45, 185, 80) direction (0, 0, -1) diameter 3.242 depth 4 tip angle 118 bodies 2
sketch "Sketch62" plane through (0, 0, 0) normal (0, 1, 0) x (-1, 0, 0)
  line L0 (133.7525, -125.611) -> (-118.245, -125.611)
  line L1 (-118.245, -125.611) -> (-118.245, -22.4859)
  line L2 (-118.245, -22.4859) -> (133.7525, -22.4859)
  line L3 (133.7525, -22.4859) -> (133.7525, -125.611)
  point P0 (0, 0)
  constraints: 8 end point, 2 parallel, 1 horizontal, 1 perpendicular
extrude "Extrusion35" cut sketch "Sketch62" along normal through all bodies 9